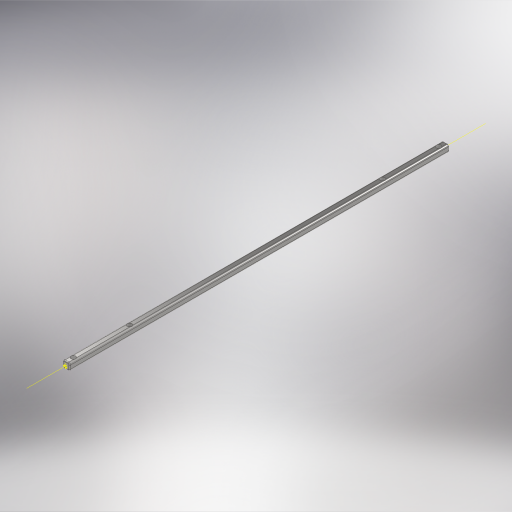
# Autodesk Inventor part: 13.5 Beam
Saved by Autodesk Inventor 2024 (Build 280153000, 153)
## iProperties
Created: 2023-08-31
Part Number: 13.5 Beam
Material: Stainless Steel
Document SubType Name: Modeling
Designer: aaron
Density: 8 g/cm^3
Appearance: Semi-Polished
Author: aaron
Autodesk Inventor part; units mm, degrees
ref_plane "YZ Plane" through (0, 0, 0) normal (1, 0, 0) x (0, 1, 0)
ref_plane "XZ Plane" through (0, 0, 0) normal (0, 1, 0) x (-1, 0, 0)
ref_plane "XY Plane" through (0, 0, 0) normal (0, 0, 1) x (1, 0, 0)
sketch "Sketch1" plane through (0, 0, 0) normal (0, 0, 1) x (1, 0, 0)
  line L0 (-3.175, 3.175) -> (3.175, 3.175)
  line L1 (3.175, 3.175) -> (3.175, -3.175)
  line L2 (3.175, -3.175) -> (-3.175, -3.175)
  line L3 (-3.175, -3.175) -> (-3.175, 3.175)
  line L4 (-3.175, 3.175) -> (3.175, -3.175) construction
  line L5 (3.175, 3.175) -> (-3.175, -3.175) construction
  point P0 (0, 0)
  dimension "d0" = 6.35
  dimension "d1" = 6.35
  constraints: 12 end point, 2 midpoint, 2 parallel, 1 horizontal, 1 perpendicular
  measures "d0" distance of L1.end L2.end
  measures "d1" distance of L0.end L1.end
extrude "Extrusion1" add sketch "Sketch1" along normal blind 342.9
sketch "Sketch2" plane through (-3.175, 3.175, 342.9) normal (0, 1, 0) x (1, 0, 0)
  circle A0 centre (3.175, 336.55) radius 2.1082
  circle A1 centre (3.175, 6.35) radius 2.1082
  line L0 (6.35, 0) -> (0, 0) projected
  line L1 (6.35, 342.9) -> (0, 342.9) projected
  circle A2 centre (3.175, 57.15) radius 2.1082
  circle A3 centre (3.175, 285.75) radius 2.1082
  point P0 (3.175, 342.9)
  dimension "d4" = 4.2164
  dimension "d5" = 4.2164
  dimension "d6" = 6.35
  dimension "d7" = 6.35
  dimension "d12" = 4.2164
  dimension "d13" = 4.2164
  dimension "d14" = 50.8
  dimension "d15" = 50.8
  constraints: 4 centre point
  measures "d4" diameter of A0
  measures "d5" diameter of A1
  measures "d6" distance from line of L0 A1.centre
  measures "d7" distance from line of A0.centre L1
  measures "d12" diameter of A2
  measures "d13" diameter of A3
  measures "d14" distance of A0.centre A3.centre
  measures "d15" distance of A1.centre A2.centre
extrude "Extrusion2" cut sketch "Sketch2" against normal blind 342.9
fillet "Fillet1" radius 1.5875 4 edges at (3.175, 3.175, 171.45) (-3.175, 3.175, 171.45) (3.175, -3.175, 171.45) (-3.175, -3.175, 171.45)
fillet "Fillet2" radius 0.7937 16 edges at (0, 3.175, 0) (-2.71, 2.71, 0) (-3.175, 0, 0) (-2.71, -2.71, 0) (0, -3.175, 0) (2.71, -2.71, 0) (3.175, 0, 0) (2.71, 2.71, 0) (2.71, 2.71, 342.9) (0, 3.175, 342.9) (-2.71, 2.71, 342.9) (-3.175, 0, 342.9) (-2.71, -2.71, 342.9) (0, -3.175, 342.9) (2.71, -2.71, 342.9) (3.175, 0, 342.9)
body "Solid1"
